Autodesk Fusion 360 part; units mm, degrees
(part 2 of 2)
  constraint coincident L69.end S24
  constraint parallel L18 L69
  constraint coincident S6.end L19.start
  constraint parallel L19 L70
extrude "Extrude6" add sketch "Sketch4" against normal blind 914.4 contours S6 L69 L70 S24
sketch "Sketch5" plane through (0, 0, 0) normal (0, -1, 0) x (1, 0, 0)
  line L0 (37033.2, 7162.8) -> (37033.2, 7618.2618)
  spline S0 degree 5 poles (37033.2, 7618.2618) (37954.428, 7611.2576) (38994.877, 7583.4187) (40033.2545, 7533.1642) (41067.7592, 7461.1483) (42096.6164, 7368.4857) (42214.8, 7357.5637) knots 0.504515 0.504515 0.504515 0.504515 0.504515 0.504515 0.55 0.555907 0.555907 0.555907 0.555907 0.555907 0.555907
  line L1 (42214.8, 7357.5637) -> (42214.8, 6856.4498)
  line L2 (42214.8, 6856.4498) -> (43129.2, 6856.4498)
  line L3 (43129.2, 6856.4498) -> (43129.2, 7266.4285)
  spline S1 degree 5 poles (43129.2, 7266.4285) (43825.0016, 7192.0589) (44874.7874, 7065.4477) (45916.0925, 6918.7228) (46947.0193, 6753.6294) (47965.7319, 6572.2462) (48310.8, 6508.7421) knots 0.565068 0.565068 0.565068 0.565068 0.565068 0.565068 0.6 0.61801 0.61801 0.61801 0.61801 0.61801 0.61801
  line L4 (48310.8, 6508.7421) -> (48310.8, 5965.9534)
  line L5 (48310.8, 5965.9534) -> (49225.2, 5965.9534)
  line L6 (49225.2, 5965.9534) -> (49225.2, 6334.6951)
  spline S2 degree 5 poles (49225.2, 6334.6951) (49650.278, 6251.1311) (50716.0208, 6033.9204) (51765.1865, 5801.4676) (52795.65, 5556.643) (53805.408, 5302.5237) (54406.8, 5146.4697) knots 0.627601 0.627601 0.627601 0.627601 0.627601 0.627601 0.65 0.684088 0.684088 0.684088 0.684088 0.684088 0.684088
  line L7 (54406.8, 5146.4697) -> (54406.8, 4569.5411)
  line L8 (54406.8, 4569.5411) -> (55321.2, 4569.5411)
  line L9 (55321.2, 4569.5411) -> (55321.2, 4904.8773)
  spline S3 degree 5 poles (55321.2, 4904.8773) (55415.9174, 4879.4147) (56375.9101, 4620.2188) (57446.8471, 4318.2729) (58486.5091, 4013.3921) (59492.5544, 3709.9309) (60382.2634, 3436.8803) (60502.8, 3399.8046) knots 0.69454 0.69454 0.69454 0.69454 0.69454 0.69454 0.7 0.75 0.757877 0.757877 0.757877 0.757877 0.757877 0.757877
  line L10 (60502.8, 3399.8046) -> (60502.8, 0)
  line L11 (60502.8, 0) -> (61417.2, 0)
  line L12 (61417.2, 0) -> (61417.2, 3116.8006)
  spline S4 degree 5 poles (61417.2, 3116.8006) (61863.0996, 2978.034) (62994.1286, 2623.9389) (64068.7047, 2284.2309) (65083.813, 1965.3744) (66037.5097, 1672.043) (66598.8, 1502.5993) knots 0.770001 0.770001 0.770001 0.770001 0.770001 0.770001 0.8 0.847529 0.847529 0.847529 0.847529 0.847529 0.847529
  line L13 (66598.8, 1502.5993) -> (66598.8, 0)
  line L14 (66598.8, 0) -> (67513.2, 0)
  line L15 (67513.2, 0) -> (67513.2, 1230.5462)
  spline S5 degree 5 poles (67513.2, 1230.5462) (67920.4439, 1111.3723) (68851.899, 844.6352) (70197.072, 484.2345) (71344.206, 225.4776) (72293.6776, 71.4215) (72883.4898, 14.4894) (73152, 0) knots 0.863462 0.863462 0.863462 0.863462 0.863462 0.863462 0.9 0.95 1 1 1 1 1 1
  line L16 (73152, 0) -> (73152, 915.9212)
  spline S6 degree 3 poles (0, 915.9214) (131.7492, 924.0422) (275.4349, 936.8365) (430.3385, 954.5737) (631.9807, 977.6627) (852.6407, 1009.1163) (1091.4063, 1049.1642) (1370.8256, 1096.0308) (1675.0543, 1154.6639) (2003.2902, 1225.1108) (2387.7561, 1307.6259) (2805.1777, 1406.3566) (3254.8084, 1520.9556) (3687.7337, 1631.2968) (4150.5377, 1756.3519) (4642.7059, 1895.3887) (5119.4939, 2030.0806) (5623.8516, 2177.9016) (6155.2434, 2337.6984) (6670.0292, 2492.5015) (7210.1951, 2658.5457) (7775.0361, 2834.2338) (8330.1548, 3006.8978) (8909.1057, 3188.8725) (9510.9669, 3378.1364) (10148.4423, 3578.5998) (10811.6233, 3787.2386) (11499.0935, 4001.1016) (12253.9288, 4235.9209) (13038.0471, 4477.0301) (13849.17, 4719.9647) (14744.4423, 4988.1025) (15672.6153, 5258.4504) (16630.1474, 5524.5468) (17641.5513, 5805.6141) (18685.7116, 6081.9109) (19757.9237, 6345.6598) (20734.1814, 6585.8053) (21733.6852, 6815.5271) (22752.5428, 7029.1759) (23672.3537, 7222.0552) (24607.9329, 7401.8264) (25556.2229, 7564.7052) (26436.32, 7715.8712) (27327.3628, 7852.4824) (28226.783, 7971.936) (29075.6964, 8084.6818) (29932.0709, 8182.1394) (30793.661, 8262.5672) (31616.2068, 8339.3503) (32443.505, 8400.6096) (33273.5419, 8445.2917) (34072.167, 8488.2829) (34873.3265, 8515.9256) (35675.1845, 8527.7544) (36468.6127, 8539.4588) (37262.722, 8535.6774) (38055.7128, 8516.4744) (38875.1791, 8496.6303) (39693.4493, 8460.3198) (40508.5709, 8408.1732) (41358.0326, 8353.8297) (42204.0738, 8282.2904) (43044.5396, 8194.8292) (43964.3855, 8099.1075) (44877.5508, 7984.314) (45781.3042, 7852.765) (46738.8463, 7713.3865) (47685.8202, 7555.205) (48619.1182, 7381.6168) (49636.7495, 7192.3432) (50638.1168, 6984.7611) (51619.4148, 6763.9051) (52702.1287, 6520.2238) (53760.4007, 6260.4022) (54789.5022, 5991.7247) (55810.6284, 5725.1294) (56803.0304, 5449.8451) (57762.5492, 5173.0777) (58630.9789, 4922.5844) (59472.4757, 4670.8911) (60284.3228, 4423.1149) (61014.7425, 4200.1904) (61721.1625, 3980.4442) (62401.8892, 3767.2754) (63034.1316, 3569.2893) (63644.2104, 3376.9821) (64231.0271, 3192.6899) (64804.6881, 3012.5293) (65356.1207, 2840.0297) (65884.5378, 2676.9357) (66421.1466, 2511.3132) (66934.0205, 2355.3936) (67422.5755, 2210.5099) (67944.1719, 2055.8277) (68438.0589, 1913.7221) (68903.7226, 1785.2281) (69393.5534, 1650.0656) (69852.1709, 1529.9574) (70278.9957, 1425.5618) (70668.6983, 1330.2457) (71031.9118, 1248.0201) (71368.0153, 1179.0625) (71662.0677, 1118.7324) (71935.3801, 1068.5561) (72187.2367, 1028.4542) (72391.7191, 995.8954) (72582.0606, 969.9782) (72757.5949, 950.525) (72898.8358, 934.8722) (73030.4952, 923.41) (73152, 915.9212) knots 0.00207705 0.00207705 0.00207705 0.00207705 0.01854804 0.01854804 0.01854804 0.03998876 0.03998876 0.03998876 0.06508013 0.06508013 0.06508013 0.09446988 0.09446988 0.09446988 0.12276769 0.12276769 0.12276769 0.1501812 0.1501812 0.1501812 0.17673804 0.17673804 0.17673804 0.20283777 0.20283777 0.20283777 0.2304819 0.2304819 0.2304819 0.26083488 0.26083488 0.26083488 0.29433681 0.29433681 0.29433681 0.3297236 0.3297236 0.3297236 0.36194355 0.36194355 0.36194355 0.39103129 0.39103129 0.39103129 0.41802728 0.41802728 0.41802728 0.44350732 0.44350732 0.44350732 0.46783269 0.46783269 0.46783269 0.4912375 0.4912375 0.4912375 0.51439626 0.51439626 0.51439626 0.53832821 0.53832821 0.53832821 0.56326839 0.56326839 0.56326839 0.59056412 0.59056412 0.59056412 0.6194844 0.6194844 0.6194844 0.65101794 0.65101794 0.65101794 0.68581042 0.68581042 0.68581042 0.72033328 0.72033328 0.72033328 0.75157881 0.75157881 0.75157881 0.77969045 0.77969045 0.77969045 0.80579986 0.80579986 0.80579986 0.83132392 0.83132392 0.83132392 0.85724366 0.85724366 0.85724366 0.88491638 0.88491638 0.88491638 0.91402526 0.91402526 0.91402526 0.94060246 0.94060246 0.94060246 0.96385449 0.96385449 0.96385449 0.98273282 0.98273282 0.98273282 0.99792296 0.99792296 0.99792296 0.99792296
  line L17 (0, 915.9214) -> (0, 0)
  spline S7 degree 5 poles (0, 0) (268.5102, 14.4894) (858.3224, 71.4215) (1807.794, 225.4776) (2954.928, 484.2346) (4300.101, 844.6352) (5231.5561, 1111.3723) (5638.8, 1230.5463) knots 0 0 0 0 0 0 0.05 0.1 0.136538 0.136538 0.136538 0.136538 0.136538 0.136538
  line L18 (5638.8, 1230.5463) -> (5638.8, 0)
  line L19 (5638.8, 0) -> (6553.2, 0)
  line L20 (6553.2, 0) -> (6553.2, 1502.5994)
  spline S8 degree 5 poles (6553.2, 1502.5994) (7114.4903, 1672.043) (8068.187, 1965.3744) (9083.2952, 2284.231) (10157.8714, 2623.9389) (11288.9004, 2978.0341) (11734.8, 3116.8007) knots 0.152471 0.152471 0.152471 0.152471 0.152471 0.152471 0.2 0.229999 0.229999 0.229999 0.229999 0.229999 0.229999
  line L21 (11734.8, 3116.8007) -> (11734.8, 0)
  line L22 (11734.8, 0) -> (12649.2, 0)
  line L23 (12649.2, 0) -> (12649.2, 3399.8047)
  spline S9 degree 5 poles (12649.2, 3399.8047) (12769.7366, 3436.8803) (13659.4456, 3709.931) (14665.4909, 4013.3922) (15705.1529, 4318.2729) (16776.0899, 4620.2189) (17736.0826, 4879.4148) (17830.8, 4904.8773) knots 0.242123 0.242123 0.242123 0.242123 0.242123 0.242123 0.25 0.3 0.30546 0.30546 0.30546 0.30546 0.30546 0.30546
  line L24 (17830.8, 4904.8773) -> (17830.8, 4569.5411)
  line L25 (17830.8, 4569.5411) -> (18745.2, 4569.5411)
  line L26 (18745.2, 4569.5411) -> (18745.2, 5146.4697)
  spline S10 degree 5 poles (18745.2, 5146.4697) (19346.592, 5302.5237) (20356.35, 5556.6431) (21386.8135, 5801.4676) (22435.9792, 6033.9205) (23501.722, 6251.1311) (23926.8, 6334.6951) knots 0.315912 0.315912 0.315912 0.315912 0.315912 0.315912 0.35 0.372399 0.372399 0.372399 0.372399 0.372399 0.372399
  line L27 (23926.8, 6334.6951) -> (23926.8, 5965.9534)
  line L28 (23926.8, 5965.9534) -> (24841.2, 5965.9534)
  line L29 (24841.2, 5965.9534) -> (24841.2, 6508.7422)
  spline S11 degree 5 poles (24841.2, 6508.7422) (25186.2681, 6572.2462) (26204.9807, 6753.6295) (27235.9075, 6918.7228) (28277.2126, 7065.4477) (29326.9984, 7192.0589) (30022.8, 7266.4285) knots 0.38199 0.38199 0.38199 0.38199 0.38199 0.38199 0.4 0.434932 0.434932 0.434932 0.434932 0.434932 0.434932
  line L30 (30022.8, 7266.4285) -> (30022.8, 6856.4498)
  line L31 (30022.8, 6856.4498) -> (30937.2, 6856.4498)
  line L32 (30937.2, 6856.4498) -> (30937.2, 7357.5637)
  spline S12 degree 5 poles (30937.2, 7357.5637) (31055.3836, 7368.4857) (32084.2408, 7461.1483) (33118.7455, 7533.1642) (34157.123, 7583.4188) (35197.572, 7611.2576) (36118.8, 7618.2618) knots 0.444093 0.444093 0.444093 0.444093 0.444093 0.444093 0.45 0.495485 0.495485 0.495485 0.495485 0.495485 0.495485
  line L33 (36118.8, 7618.2618) -> (36118.8, 7162.8)
  line L34 (36118.8, 7162.8) -> (37033.2, 7162.8)
sketch "Sketch6" plane through (0, 0, 0) normal (0, -1, 0) x (1, 0, 0)
mirror "Mirror1" about plane through (36576, 4267.2, 4726.9675) normal (0, 1, 0) of bodies 1 merged
chamfer "Chamfer2" distance 9753.6 distance2 914.4 1 edges at (73152, 4267.2, 915.9212) measured on face at (3170.0003, 3759.2, 1499.432)
chamfer "Chamfer3" distance 914.4 distance2 9753.6 1 edges at (0, 4267.2, 915.9214) measured on face at (0, 3149.6, 305.3071)
